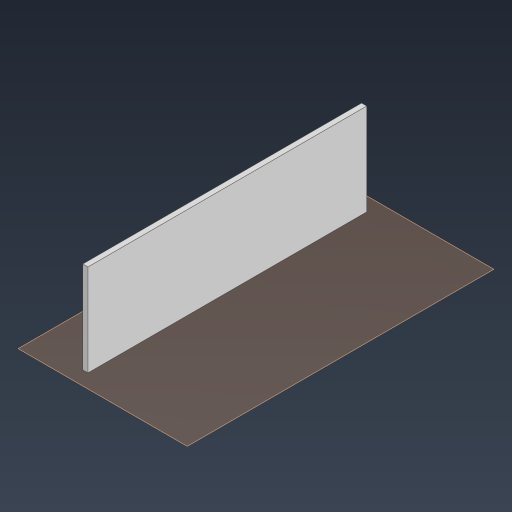
# Autodesk Inventor part: pcb-holder-right
Saved by Autodesk Inventor 2023 (Build 270158000, 158)
## iProperties
Created: 2025-04-06
Part Number: pcb-holder-right
Material: Generic
Document SubType Name: Modeling
Designer: szymo
Density: 1 g/cm^3
Appearance: Default
Author: szymo
Autodesk Inventor part; units mm, degrees
ref_plane "YZ Plane" through (0, 0, 0) normal (1, 0, 0) x (0, 1, 0)
ref_plane "XZ Plane" through (0, 0, 0) normal (0, 1, 0) x (-1, 0, 0)
ref_plane "XY Plane" through (0, 0, 0) normal (0, 0, 1) x (1, 0, 0)
ref_plane "Work Plane1" through (-14.8376, -17.7, 26.9) normal (0, 1, 0) x (0, 0, -1)
sketch "Sketch1" plane through (-14.8376, -17.7, 26.9) normal (0, 1, 0) x (0, 0, -1)
  circle A0 centre (-11.6, -9.9714) radius 12.5 projected
  circle A1 centre (13.9, -9.9714) radius 12.5 projected
  line L0 (26.9, 12.8624) -> (26.9, -14.8376) projected
  line L1 (16.8986, 12.8624) -> (26.9, 12.8624) projected
  arc A2 (16.8986, 12.8624) -> (6.7153, 12.8624) centre (11.8069, 7.2876) ccw projected
  line L2 (-26.9, 12.8624) -> (6.7153, 12.8624) projected
  line L3 (-26.9, -14.8376) -> (-26.9, 12.8624) projected
  line L4 (26.9, -14.8376) -> (-26.9, -14.8376) projected
  circle A3 centre (13.9, -9.9714) radius 4.2 projected
  circle A4 centre (-11.6, -9.9714) radius 4.2 projected
  line L5 (-26.9, 5.5286) -> (26.9, 5.5286)
  line L6 (-26.9, 6.5286) -> (26.9, 6.5286)
  dimension "d0" = 3
  dimension "d1" = 1
  constraints: 4 end point, 4 point on line, 2 perpendicular
  measures "d0" distance edge to line of A0 L5
  measures "d1" distance between parallel lines of L6 L5
ref_plane "Work Plane2" through (-30.4312, 0, 53.8) normal (0, 1, 0) x (0, 0, 1)
extrude "Extrusion1" add sketch "Sketch1" along normal up to surface (17.7 mm away) contours L3 L6 L0 L5
body "Solid1"
